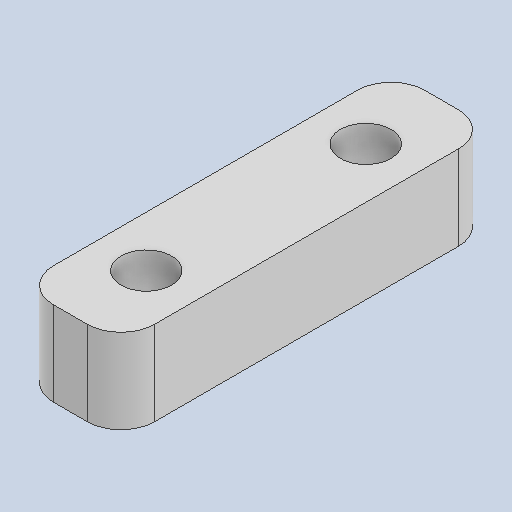
# Autodesk Inventor part: cable_holder
Saved by Autodesk Inventor 2025 (Build 290162000, 162)
## iProperties
Created: 2025-08-20
Part Number: cable_holder
Material: Generic
Document SubType Name: Modeling
Designer: Pravoslav
Density: 1 g/cm^3
Appearance: Default
Author: Pravoslav
Autodesk Inventor part; units mm, degrees
ref_plane "YZ Plane" through (0, 0, 0) normal (1, 0, 0) x (0, 1, 0)
ref_plane "XZ Plane" through (0, 0, 0) normal (0, 1, 0) x (-1, 0, 0)
ref_plane "XY Plane" through (0, 0, 0) normal (0, 0, 1) x (1, 0, 0)
sketch "Sketch1" plane through (0, 0, 0) normal (0, 1, 0) x (-1, 0, 0)
  circle A0 centre (0, 6.5) radius 1.5
  circle A1 centre (0, -6.5) radius 1.5
  line L0 (3, 11) -> (-3, 11)
  line L1 (-3, 11) -> (-3, -11)
  line L2 (-3, -11) -> (3, -11)
  line L3 (3, -11) -> (3, 11)
  line L4 (3, 11) -> (-3, -11) construction
  line L5 (-3, 11) -> (3, -11) construction
  point P0 (0, 0)
  dimension "d0" = 3
  dimension "d1" = 3
  dimension "d2" = 13
  dimension "d3" = 6.5
  dimension "d4" = 6
  dimension "d5" = 22
  constraints: 12 end point, 2 centre point, 2 midpoint, 2 parallel, 1 horizontal, 1 perpendicular
  measures "d0" diameter of A0
  measures "d1" diameter of A1
  measures "d2" distance of A1.centre A0.centre
  measures "d3" distance of point (0, 0) A1.centre
  measures "d4" distance of L2.end L1.end
  measures "d5" distance of L1.end L0.end
extrude "Extrusion1" add sketch "Sketch1" along normal blind 5
fillet "Fillet1" radius 2 4 edges at (-3, 2.5, 11) (3, 2.5, 11) (3, 2.5, -11) (-3, 2.5, -11)
body "Solid1"
